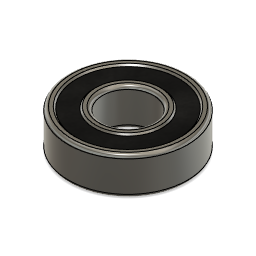
Bearing v4 (Autodesk Fusion 360 design; units mm, degrees)
Autodesk Fusion 360 part; units mm, degrees
sketch "Basis" plane through (0, 0, 0) normal (0, 1, 0) x (1, 0, 0)
  circle A0 centre (0, 0) radius 7.5
  circle A1 centre (0, 0) radius 17.5
  circle A2 centre (0, 0) radius 10
  dimension "d1" = 15
  dimension "d3" = 35
  dimension "d7" = 20
  constraint coincident A0.centre A1.centre
  constraint concentric A1 A2
  measures "d1" diameter of A0
  measures "d3" diameter of A1
  measures "d7" diameter of A2
extrude "Extrude1" add sketch "Basis" along normal blind 11 contours A1 | A2
sketch "Edges" plane through (0, 0, 0) normal (0, 1, 0) x (1, 0, 0)
  circle A0 centre (0, 0) radius 7.5
  circle A1 centre (0, 0) radius 17.5
  circle A2 centre (0, 0) radius 10
  circle A3 centre (0, 0) radius 15
  dimension "d20" = 2.5
  dimension "d21" = -2.5
extrude "Extrude2" cut sketch "Edges" along normal blind 0.5 contours A3
chamfer "Chamfer1" distance 0.5 angle 45 2 edges at (-9.3233, 0, -3.6162) (-13.9849, 0, 5.4242)
fillet "Fillet1" radius 1 2 edges at (-6.9925, 0, -2.7121) (-16.3157, 0, 6.3283)
ref_plane "WorkPlane1" through (0, 5.5, 0) normal (0, -1, 0) x (-1, 0, 0)
mirror "Mirror1" about plane through (0, 5.5, 0) normal (0, -1, 0) of "Extrude2", "Chamfer1", "Fillet1"
named bodies: "Bearing"
